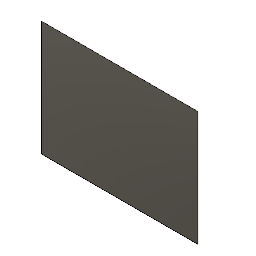
not subtracivly made v1 v1 (Autodesk Fusion 360 design; units mm, degrees)
Autodesk Fusion 360 part; units mm, degrees
sketch "Sketch1" plane through (0, 0, 0) normal (0, 0, 1) x (1, 0, 0)
  line L0 (0, 0) -> (-75, 0)
  line L1 (-75, 0) -> (-75, 50)
  line L2 (-75, 50) -> (0, 50)
  line L3 (0, 50) -> (0, 0)
extrude "Extrude1" add sketch "Sketch1" along normal blind 10 draft 45
